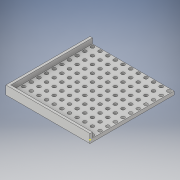
# Autodesk Inventor part: dontlossethis
Saved by Autodesk Inventor 2018 (Build 220112000, 112)
## iProperties
Created: 2018-05-07
Part Number: dontlossethis
Material: Generic
Document SubType Name: Modeling
Designer: 4070609
Density: 1 g/cm^3
Appearance: Default
Author: 4070609
Autodesk Inventor part; units mm, degrees
ref_plane "YZ Plane" through (0, 0, 0) normal (1, 0, 0) x (0, 1, 0)
ref_plane "XZ Plane" through (0, 0, 0) normal (0, 1, 0) x (-1, 0, 0)
ref_plane "XY Plane" through (0, 0, 0) normal (0, 0, 1) x (1, 0, 0)
sketch "Sketch1" plane through (0, 0, 0) normal (0, 1, 0) x (-1, 0, 0)
  line L0 (0, 0) -> (48.4, 0)
  line L1 (48.4, 0) -> (48.4, -48.4)
  line L2 (48.4, -48.4) -> (0, -48.4)
  line L3 (0, -48.4) -> (0, 0)
  dimension "d0" = 48.4
  dimension "d1" = 48.4
  constraints: 8 end point, 2 parallel, 1 horizontal, 1 perpendicular
  measures "d0" distance of L1.end L2.end
  measures "d1" distance of L0.end L1.end
extrude "Extrusion1" add sketch "Sketch1" along normal blind 2
sketch "Sketch2" plane through (0, 2, 0) normal (0, 1, 0) x (1, 0, 0)
  line L0 (-48.4, 0) -> (0, 0) projected
  line L1 (0, 0) -> (0, 48.4) projected
  line L2 (-48.4, 0) -> (0, 0)
  line L3 (0, 0) -> (0, 1.4)
  line L4 (0, 1.4) -> (-48.4, 1.4)
  line L5 (-48.4, 1.4) -> (-48.4, 0)
  line L6 (-48.4, 0) -> (-47, 0)
  line L7 (-47, 0) -> (-47, 48.4)
  line L8 (-47, 48.4) -> (-48.4, 48.4)
  line L9 (-48.4, 48.4) -> (-48.4, 0)
  dimension "d4" = 1.4
  dimension "d5" = 1.4
  constraints: 16 end point, 4 parallel, 2 horizontal, 2 perpendicular, 1 point on line
  measures "d4" distance of L3.end L2.end
  measures "d5" distance of L8.end L7.end
extrude "Extrusion2" add sketch "Sketch2" along normal blind 3
sketch "Sketch3" plane through (0, 2, 0) normal (0, 1, 0) x (1, 0, 0)
  point P0 (0, 0)
sketch "Sketch4" plane through (0, 2, 0) normal (0, 1, 0) x (1, 0, 0)
  point P0 (0, 0)
sketch "Sketch5" plane through (0, 2, 0) normal (0, 1, 0) x (1, 0, 0)
  line L0 (-48.4, 0) -> (-48.4, 48.4) projected
  line L1 (-48.4, 0) -> (-45.5, 0)
  line L2 (-45.5, 0) -> (-45.5, 2.9)
  line L3 (-45.5, 2.9) -> (-48.4, 2.9)
  line L4 (-48.4, 2.9) -> (-48.4, 0)
  circle A0 centre (-45.5, 2.9) radius 1
  line L5 (-45.5, 4.4) -> (-45.5, 7.3)
  circle A1 centre (-45.5, 7.3) radius 1
  line L6 (-45.5, 8.8) -> (-45.5, 11.7)
  circle A2 centre (-45.5, 11.7) radius 1
  line L7 (-45.5, 13.2) -> (-45.5, 16.1)
  circle A3 centre (-45.5, 16.1) radius 1
  line L8 (-45.5, 17.6) -> (-45.5, 20.5)
  circle A4 centre (-45.5, 20.5) radius 1
  line L9 (-45.5, 22) -> (-45.5, 24.9)
  circle A5 centre (-45.5, 24.9) radius 1
  line L10 (-45.5, 26.4) -> (-45.5, 29.3)
  circle A6 centre (-45.5, 29.3) radius 1
  line L11 (-45.5, 30.8) -> (-45.5, 33.7)
  circle A7 centre (-45.5, 33.7) radius 1
  line L12 (-45.5, 35.2) -> (-45.5, 38.1)
  circle A8 centre (-45.5, 38.1) radius 1
  line L13 (-45.5, 39.6) -> (-45.5, 42.5)
  circle A9 centre (-45.5, 42.5) radius 1
  line L14 (-45.5, 44) -> (-45.5, 46.9)
  circle A10 centre (-45.5, 46.9) radius 1
  line L15 (-38.0114, 1.4) -> (-29.4522, 1.4)
  line L16 (-47, 1.4) -> (0, 1.4) projected
  circle A11 centre (-41.1, 2.9) radius 1
  circle A12 centre (-41.1, 7.3) radius 1
  circle A13 centre (-41.1, 11.7) radius 1
  circle A14 centre (-41.1, 16.1) radius 1
  circle A15 centre (-41.1, 20.5) radius 1
  circle A16 centre (-41.1, 24.9) radius 1
  circle A17 centre (-41.1, 29.3) radius 1
  circle A18 centre (-41.1, 33.7) radius 1
  circle A19 centre (-41.1, 38.1) radius 1
  circle A20 centre (-41.1, 42.5) radius 1
  circle A21 centre (-41.1, 46.9) radius 1
  circle A22 centre (-36.7, 2.9) radius 1
  circle A23 centre (-36.7, 7.3) radius 1
  circle A24 centre (-36.7, 11.7) radius 1
  circle A25 centre (-36.7, 16.1) radius 1
  circle A26 centre (-36.7, 20.5) radius 1
  circle A27 centre (-36.7, 24.9) radius 1
  circle A28 centre (-36.7, 29.3) radius 1
  circle A29 centre (-36.7, 33.7) radius 1
  circle A30 centre (-36.7, 38.1) radius 1
  circle A31 centre (-36.7, 42.5) radius 1
  circle A32 centre (-36.7, 46.9) radius 1
  circle A33 centre (-32.3, 2.9) radius 1
  circle A34 centre (-32.3, 7.3) radius 1
  circle A35 centre (-32.3, 11.7) radius 1
  circle A36 centre (-32.3, 16.1) radius 1
  circle A37 centre (-32.3, 20.5) radius 1
  circle A38 centre (-32.3, 24.9) radius 1
  circle A39 centre (-32.3, 29.3) radius 1
  circle A40 centre (-32.3, 33.7) radius 1
  circle A41 centre (-32.3, 38.1) radius 1
  circle A42 centre (-32.3, 42.5) radius 1
  circle A43 centre (-32.3, 46.9) radius 1
  circle A44 centre (-27.9, 2.9) radius 1
  circle A45 centre (-27.9, 7.3) radius 1
  circle A46 centre (-27.9, 11.7) radius 1
  circle A47 centre (-27.9, 16.1) radius 1
  circle A48 centre (-27.9, 20.5) radius 1
  circle A49 centre (-27.9, 24.9) radius 1
  circle A50 centre (-27.9, 29.3) radius 1
  circle A51 centre (-27.9, 33.7) radius 1
  circle A52 centre (-27.9, 38.1) radius 1
  circle A53 centre (-27.9, 42.5) radius 1
  circle A54 centre (-27.9, 46.9) radius 1
  circle A55 centre (-23.5, 2.9) radius 1
  circle A56 centre (-23.5, 7.3) radius 1
  circle A57 centre (-23.5, 11.7) radius 1
  circle A58 centre (-23.5, 16.1) radius 1
  circle A59 centre (-23.5, 20.5) radius 1
  circle A60 centre (-23.5, 24.9) radius 1
  circle A61 centre (-23.5, 29.3) radius 1
  circle A62 centre (-23.5, 33.7) radius 1
  circle A63 centre (-23.5, 38.1) radius 1
  circle A64 centre (-23.5, 42.5) radius 1
  circle A65 centre (-23.5, 46.9) radius 1
  circle A66 centre (-19.1, 2.9) radius 1
  circle A67 centre (-19.1, 7.3) radius 1
  circle A68 centre (-19.1, 11.7) radius 1
  circle A69 centre (-19.1, 16.1) radius 1
  circle A70 centre (-19.1, 20.5) radius 1
  circle A71 centre (-19.1, 24.9) radius 1
  circle A72 centre (-19.1, 29.3) radius 1
  circle A73 centre (-19.1, 33.7) radius 1
  circle A74 centre (-19.1, 38.1) radius 1
  circle A75 centre (-19.1, 42.5) radius 1
  circle A76 centre (-19.1, 46.9) radius 1
  circle A77 centre (-14.7, 2.9) radius 1
  circle A78 centre (-14.7, 7.3) radius 1
  circle A79 centre (-14.7, 11.7) radius 1
  circle A80 centre (-14.7, 16.1) radius 1
  circle A81 centre (-14.7, 20.5) radius 1
  circle A82 centre (-14.7, 24.9) radius 1
  circle A83 centre (-14.7, 29.3) radius 1
  circle A84 centre (-14.7, 33.7) radius 1
  circle A85 centre (-14.7, 38.1) radius 1
  circle A86 centre (-14.7, 42.5) radius 1
  circle A87 centre (-14.7, 46.9) radius 1
  circle A88 centre (-10.3, 2.9) radius 1
  circle A89 centre (-10.3, 7.3) radius 1
  circle A90 centre (-10.3, 11.7) radius 1
  circle A91 centre (-10.3, 16.1) radius 1
  circle A92 centre (-10.3, 20.5) radius 1
  circle A93 centre (-10.3, 24.9) radius 1
  circle A94 centre (-10.3, 29.3) radius 1
  circle A95 centre (-10.3, 33.7) radius 1
  circle A96 centre (-10.3, 38.1) radius 1
  circle A97 centre (-10.3, 42.5) radius 1
  circle A98 centre (-10.3, 46.9) radius 1
  circle A99 centre (-5.9, 2.9) radius 1
  circle A100 centre (-5.9, 7.3) radius 1
  circle A101 centre (-5.9, 11.7) radius 1
  circle A102 centre (-5.9, 16.1) radius 1
  circle A103 centre (-5.9, 20.5) radius 1
  circle A104 centre (-5.9, 24.9) radius 1
  circle A105 centre (-5.9, 29.3) radius 1
  circle A106 centre (-5.9, 33.7) radius 1
  circle A107 centre (-5.9, 38.1) radius 1
  circle A108 centre (-5.9, 42.5) radius 1
  circle A109 centre (-5.9, 46.9) radius 1
  circle A110 centre (-1.5, 2.9) radius 1
  circle A111 centre (-1.5, 7.3) radius 1
  circle A112 centre (-1.5, 11.7) radius 1
  circle A113 centre (-1.5, 16.1) radius 1
  circle A114 centre (-1.5, 20.5) radius 1
  circle A115 centre (-1.5, 24.9) radius 1
  circle A116 centre (-1.5, 29.3) radius 1
  circle A117 centre (-1.5, 33.7) radius 1
  circle A118 centre (-1.5, 38.1) radius 1
  circle A119 centre (-1.5, 42.5) radius 1
  circle A120 centre (-1.5, 46.9) radius 1
  point P0 (0, 0)
  dimension "d8" = 2.9
  dimension "d9" = 2.9
  dimension "d10" = 2
  dimension "d13" = 4.4
  dimension "d20" = 4.4
  constraints: 121 centre point, 30 end point, 11 coincident, 2 horizontal, 2 parallel, 1 perpendicular, 1 point on line, 1 vertical, 270 other
  measures "d8" distance of L3.end L2.end
  measures "d9" distance of L1.end L2.end
  measures "d10" diameter of A0
  measures "d13" distance of L1.end L5.start
  measures "d20" distance of A0.centre A11.centre
extrude "Extrusion3" cut sketch "Sketch5" against normal blind 2 contours A0 L2 L3 | L3 L2 A0 | A1 | A2 | A3 | A4 | A5 | A6 | A7 | A8 | A9 | A10 | A11 | A12 | A13 | A14 | A15 | A16 | A17 | A18 | A19 | A20 | A21 | A22 | A23 | A24 | A25 | A26 | A27 | A28 | A29 | A30 | A31 | A32 | A33 | A34 | A35 | A36 | A37 | A38 | A39 | A40 | A41 | A42 | A43 | A44 | A45 | A46 | A47 | A48 | A49 | A50 | A51 | A52 | A53 | A54 | A55 | A56 | A57 | A58 | A59 | A60 | A61 | A62 | A63 | A64 | A65 | A66 | A67 | A68 | A69 | A70 | A71 | A72 | A73 | A74 | A75 | A76 | A77 | A78 | A79 | A80 | A81 | A82 | A83 | A84 | A85 | A86 | A87 | A88 | A89 | A90 | A91 | A92 | A93 | A94 | A95 | A96 | A97 | A98 | A99 | A100 | A101 | A102 | A103 | A104 | A105 | A106 | A107 | A108 | A109 | A110 | A111 | A112 | A113 | A114 | A115 | A116 | A117 | A118 | A119 | A120
fillet "Fillet1" radius 0.4 121 edges at (-46.5, 0, -2.9) (-42.1, 0, -2.9) (-37.7, 0, -2.9) (-33.3, 0, -2.9) (-28.9, 0, -2.9) (-24.5, 0, -2.9) (-20.1, 0, -2.9) (-15.7, 0, -2.9) (-11.3, 0, -2.9) (-6.9, 0, -2.9) (-2.5, 0, -2.9) (-2.5, 0, -7.3) (-6.9, 0, -7.3) (-11.3, 0, -7.3) (-15.7, 0, -7.3) (-20.1, 0, -7.3) (-24.5, 0, -7.3) (-28.9, 0, -7.3) (-33.3, 0, -7.3) (-37.7, 0, -7.3) (-42.1, 0, -7.3) (-46.5, 0, -7.3) (-46.5, 0, -11.7) (-42.1, 0, -11.7) (-37.7, 0, -11.7) (-33.3, 0, -11.7) (-28.9, 0, -11.7) (-24.5, 0, -11.7) (-20.1, 0, -11.7) (-15.7, 0, -11.7) (-11.3, 0, -11.7) (-6.9, 0, -11.7) (-2.5, 0, -11.7) (-2.5, 0, -16.1) (-6.9, 0, -16.1) (-11.3, 0, -16.1) (-15.7, 0, -16.1) (-20.1, 0, -16.1) (-24.5, 0, -16.1) (-28.9, 0, -16.1) (-33.3, 0, -16.1) (-37.7, 0, -16.1) (-42.1, 0, -16.1) (-46.5, 0, -16.1) (-46.5, 0, -20.5) (-42.1, 0, -20.5) (-37.7, 0, -20.5) (-33.3, 0, -20.5) (-28.9, 0, -20.5) (-24.5, 0, -20.5) (-20.1, 0, -20.5) (-15.7, 0, -20.5) (-11.3, 0, -20.5) (-6.9, 0, -20.5) (-2.5, 0, -20.5) (-2.5, 0, -24.9) (-6.9, 0, -24.9) (-11.3, 0, -24.9) (-15.7, 0, -24.9) (-20.1, 0, -24.9) (-24.5, 0, -24.9) (-28.9, 0, -24.9) (-33.3, 0, -24.9) (-37.7, 0, -24.9) (-42.1, 0, -24.9) (-46.5, 0, -24.9) (-46.5, 0, -29.3) (-42.1, 0, -29.3) (-37.7, 0, -29.3) (-33.3, 0, -29.3) (-28.9, 0, -29.3) (-24.5, 0, -29.3) (-20.1, 0, -29.3) (-15.7, 0, -29.3) (-11.3, 0, -29.3) (-6.9, 0, -29.3) (-2.5, 0, -29.3) (-2.5, 0, -33.7) (-6.9, 0, -33.7) (-11.3, 0, -33.7) (-15.7, 0, -33.7) (-20.1, 0, -33.7) (-24.5, 0, -33.7) (-28.9, 0, -33.7) (-33.3, 0, -33.7) (-37.7, 0, -33.7) (-42.1, 0, -33.7) (-46.5, 0, -33.7) (-46.5, 0, -38.1) (-42.1, 0, -38.1) (-37.7, 0, -38.1) (-33.3, 0, -38.1) (-28.9, 0, -38.1) (-24.5, 0, -38.1) (-20.1, 0, -38.1) (-15.7, 0, -38.1) (-11.3, 0, -38.1) (-6.9, 0, -38.1) (-2.5, 0, -38.1) (-2.5, 0, -42.5) (-6.9, 0, -42.5) (-11.3, 0, -42.5) (-15.7, 0, -42.5) (-20.1, 0, -42.5) (-24.5, 0, -42.5) (-28.9, 0, -42.5) (-33.3, 0, -42.5) (-37.7, 0, -42.5) (-42.1, 0, -42.5) (-46.5, 0, -42.5) (-46.5, 0, -46.9) (-42.1, 0, -46.9) (-37.7, 0, -46.9) (-33.3, 0, -46.9) (-28.9, 0, -46.9) (-24.5, 0, -46.9) (-20.1, 0, -46.9) (-15.7, 0, -46.9) (-11.3, 0, -46.9) (-6.9, 0, -46.9) (-2.5, 0, -46.9)
body "Solid1"
